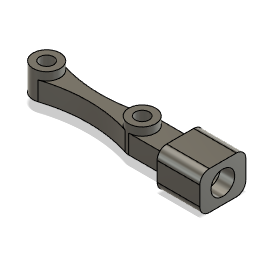
sensor_servo_mounting (Autodesk Fusion 360 design; units mm, degrees)
Autodesk Fusion 360 part; units mm, degrees
sketch "Arm" plane through (0, 0, 0) normal (0, 1, 0) x (1, 0, 0)
  line L0 (0, 2.85) -> (-35, 2.85)
  line L1 (-35, 2.85) -> (-35, -2.85)
  line L2 (-35, -2.85) -> (0, -2.85)
  line L3 (0, -2.85) -> (0, 2.85)
  line L4 (-35, 0) -> (0, 0) construction
  circle A0 centre (-32.15, 0) radius 1.7
  circle A1 centre (-32.15, 0) radius 2.35 construction
  circle A2 centre (-32.15, 0) radius 2.85
  line L5 (-30.45, 0) -> (-30.45, 2.85) construction
  line L6 (-22.075, 0) -> (-22.075, 2.85) construction
  circle A3 centre (-12, 0) radius 2.85
  line L7 (-29.5888, 1.25) -> (-14.5612, 1.25) construction
  arc A4 (-31.2671, 2.7098) -> (-12.8829, 2.7098) centre (-22.075, 30.9205) ccw
  arc A5 (-12.8829, -2.7098) -> (-31.2671, -2.7098) centre (-22.075, -30.9205) ccw
  circle A6 centre (-32.15, 0) radius 1.475
  circle A7 centre (-12, 0) radius 1.475
  dimension "d5" = 35
  dimension "d64" = 5.7
  dimension "d65" = 3.4
  dimension "d66" = 4.7
  dimension "d67" = 8.375
  dimension "d68" = 1.25
  dimension "d69" = 2.95
  constraint horizontal L0
  constraint vertical L1
  constraint horizontal L2
  constraint vertical L3
  constraint midpoint L1 L4.start
  constraint midpoint L3 L4.end
  constraint coincident L4.end origin
  constraint coincident L4 A0.centre
  constraint concentric A0 A1
  constraint tangent L0 A2
  constraint tangent L1 A2
  constraint tangent L2 A2
  constraint coincident A0.centre A1.centre
  constraint coincident A0 L5.start
  constraint coincident L4 L5.start
  constraint coincident L0 L5.end
  constraint perpendicular L0 L5
  constraint coincident L4 L6.start
  constraint coincident L0 L6.end
  constraint perpendicular L0 L6
  constraint symmetric A2 L6 A3
  constraint coincident A2 L7.start
  constraint coincident A3 L7.end
  constraint perpendicular L6 L7
  constraint coincident A3 A4.end
  constraint coincident A2 A4.start
  constraint tangent A2 A4
  constraint tangent A3 A4
  constraint tangent L7 A4
  constraint symmetric L4 A4.start A5.end
  constraint symmetric L4 A4.end A5.start
  constraint symmetric L4 A4 A5
  constraint concentric A0 A6
  constraint symmetric L6 A6 A7
  measures "d5" distance of L0.start L0.end
  measures "d64" distance of L0.end L1.end
  measures "d65" diameter of A0
  measures "d66" diameter of A1
  measures "d67" distance of L5 L6
  measures "d68" distance of L4 L7
  measures "d69" diameter of A6
extrude "Extrude1" add sketch "Arm" along normal mid plane 4 contours L0 L2 L3 A3 | A3 | A2 | A2 A3 A4 A5 | A0 | A6 | A7 makes body 1
extrude "Extrude6" add sketch "Arm" along normal blind 1.7 from surface at 2 contours A3 | A2 | A0 bodies 1
extrude "Extrude7" cut sketch "Arm" along normal up to surface (3.7 mm away) contours A6 | A7 bodies 1
sketch "Servo" plane through (0, 0, 0) normal (1, 0, 0) x (0, 0, -1)
  line L0 (2.85, -2) -> (2.85, 2)
  line L1 (2.85, 2) -> (-2.85, 2)
  line L2 (-2.85, 2) -> (-2.85, -2)
  line L3 (-2.85, -2) -> (2.85, -2)
  line L4 (-4.85, -4) -> (4.85, -4)
  line L5 (4.85, -4) -> (4.85, 4)
  line L6 (4.85, 4) -> (-4.85, 4)
  line L7 (-4.85, 4) -> (-4.85, -4)
  circle A0 centre (0, 0) radius 2.5
  circle A1 centre (0, 0) radius 1.2
  line L8 (2.85, -2) -> (2.85, 2)
  line L9 (2.85, 2) -> (-2.85, 2)
  line L10 (-2.85, 2) -> (-2.85, -2)
  line L11 (-2.85, -2) -> (2.85, -2)
  circle A2 centre (0, 0) radius 2.2
  dimension "d44" = 2
  dimension "d45" = 5
  dimension "d46" = 2.4
  dimension "d61" = 4.4
  constraint coincident A0.centre A1.centre
  measures "d45" diameter of A0
  measures "d46" diameter of A1
  measures "d61" diameter of A2
extrude "Screw head hole in arm" cut sketch "Servo" against normal blind 1.4 contours L0 L1 L3 A0 L8 L9 L11 | L1 L3 A0 L9 L11 A2 | L1 L3 L9 L11 A2 | L1 L3 A0 L9 L11 A2 | L1 L2 L3 A0 L9 L10 L11 | A1 bodies 1
extrude "Extrude9" add sketch "Servo" against normal blind 4 separate body contours L3 A0 L11 A2 | L1 A0 L9 A2 | L4 L5 L6 L7 makes body 2
extrude "Extrude10" add sketch "Servo" along normal blind 1 contours L0 L1 L3 A0 L8 L9 L11 | L3 A0 L11 A2 | L1 L3 A0 L9 L11 A2 | L1 A0 L9 A2 | L3 L11 A2 | L1 L3 L9 L11 A2 | L1 L3 A0 L9 L11 A2 | L1 L2 L3 A0 L9 L10 L11 | L1 L9 A2 | L4 L5 L6 L7 bodies 2
extrude "Extrude11" add sketch "Servo" along normal blind 4 from surface at 1 contours L0 L1 L3 A0 L8 L9 L11 | L1 L2 L3 A0 L9 L10 L11 | L4 L5 L6 L7 bodies 2
move_face "OffsetFaces1" offset -0.1 4 faces at (-1.3333, -0.6667, -2.85) (-1.3333, 2, -2.2055) (-1.3333, 0.6667, 2.85) (-1.3333, -2, 2.2055) on bodies 2
chamfer "Chamfer2" distance 1 angle 45 1 edges at (1, -0.904, 2.3308) on bodies 2
fillet "Fillet3" radius 2 4 edges at (0.5, 4, 4.85) (0.5, -4, 4.85) (0.5, -4, -4.85) (0.5, 4, -4.85) on bodies 2
equation "d5 = length - screw_wall - servo_height"
equation "d10 = height"
equation "length = 40 mm"
equation "height = 2 mm"
equation "servo_diameter = 5 mm"
equation "servo_screw_diameter = 2.4 mm"
equation "servo_height = 4 mm"
equation "d45 = servo_diameter"
equation "d46 = servo_screw_diameter"
equation "connector_length = 4 mm"
equation "d48 = -connector_length"
equation "d53 = servo_height"
equation "screw_wall = 1 mm"
equation "d61 = servo_screw_head_diameter"
equation "servo_screw_head_diameter = 4.4 mm"
equation "d67 = ( 16.75 / 2 ) * 1 mm"
named bodies: "Sensor handle", "Servo handle"
